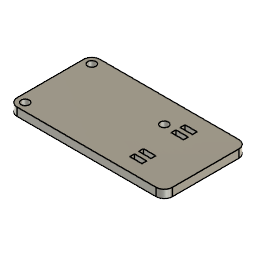
Arnes v1 (Autodesk Fusion 360 design; units mm, degrees)
Autodesk Fusion 360 part; units mm, degrees
(part 1 of 2)
sketch "Boceto1" plane through (0, 0, 0) normal (0, 0, 1) x (1, 0, 0)
  arc A0 (2, 20.32) -> (0, 18.32) centre (2, 18.32) ccw
  arc A1 (0, 2) -> (2, 0) centre (2, 2) ccw
  arc A2 (36.08, 0) -> (38.08, 2) centre (36.08, 2) ccw
  line L0 (38.08, 2) -> (38.08, 18.32)
  line L1 (36.08, 20.32) -> (2, 20.32)
  arc A3 (38.08, 18.32) -> (36.08, 20.32) centre (36.08, 18.32) ccw
  line L2 (2, 0) -> (36.08, 0)
  line L3 (0, 18.32) -> (0, 2)
  line L4 (25.2, 8.47, 1.57) -> (25.2, 7.99, 1.57)
  line L5 (25.2, 7.99, 1.57) -> (25.6, 7.99, 1.57)
  line L6 (25.6, 7.99, 1.57) -> (25.6, 8.47, 1.57)
  line L7 (25.6, 8.47, 1.57) -> (25.2, 8.47, 1.57)
  line L8 (25.2, 9.79, 1.57) -> (25.2, 9.31, 1.57)
  line L9 (25.6, 9.31, 1.57) -> (25.6, 9.79, 1.57)
  line L10 (25.6, 9.79, 1.57) -> (25.2, 9.79, 1.57)
  line L11 (25.2, 9.31, 1.57) -> (25.6, 9.31, 1.57)
  line L12 (24.511, 9.525, 1.57) -> (24.511, 7.9796, 1.57)
  line L13 (25.957, 8.1792, 1.57) -> (26.3634, 8.1792, 1.57)
  line L14 (25.957, 9.574, 1.57) -> (25.957, 8.1792, 1.57)
  line L15 (24.511, 7.9796, 1.57) -> (24.9174, 7.9796, 1.57)
  line L16 (26.3634, 9.574, 1.57) -> (25.957, 9.574, 1.57)
  line L17 (24.9174, 7.9796, 1.57) -> (24.9174, 9.525, 1.57)
  line L18 (26.3634, 8.1792, 1.57) -> (26.3634, 9.574, 1.57)
  line L19 (24.9174, 9.525, 1.57) -> (24.511, 9.525, 1.57)
  line L20 (25.85, 8.24, 1.571) -> (25.85, 9.54, 1.571)
  line L21 (24.95, 8.24, 1.571) -> (25.85, 8.24, 1.571)
  line L22 (24.95, 9.54, 1.571) -> (24.95, 8.24, 1.571)
  line L23 (25.85, 9.54, 1.571) -> (24.95, 8.24, 1.571)
  line L24 (25.85, 8.24, 1.571) -> (24.95, 9.54, 1.571)
  line L25 (25.85, 9.54, 1.571) -> (24.95, 9.54, 1.571)
  line L26 (25.4, 9.44, 1.72) -> (25.4, 9.44, 1.57)
  line L27 (25.4, 8.04, 1.57) -> (25.4, 8.04, 1.72)
  line L28 (25.4, 8.04, 1.72) -> (25.4, 8.34, 1.72)
  line L29 (25.4, 8.34, 1.72) -> (25.4, 8.34, 1.57)
  line L30 (25.4, 8.04, 1.72) -> (25.4, 8.34, 1.57)
  line L31 (25.4, 9.44, 1.57) -> (25.4, 9.74, 1.57)
  line L32 (25.4, 9.74, 1.57) -> (25.4, 9.74, 1.72)
  line L33 (25.4, 9.74, 1.72) -> (25.4, 9.44, 1.72)
  line L34 (25.4, 9.74, 1.72) -> (25.4, 9.44, 1.57)
  line L35 (25.4, 8.34, 1.57) -> (25.4, 8.04, 1.57)
  line L36 (25.4, 8.34, 1.72) -> (25.4, 8.04, 1.57)
  line L37 (25.4, 9.44, 1.72) -> (25.4, 9.74, 1.57)
  line L38 (25.02, 9.47, 2.27) -> (25.02, 9.21, 2.27)
  line L39 (25.4, 8.89, 2.27) -> (26.4, 8.89, 2.27)
  line L40 (25.78, 9.47, 2.27) -> (25.02, 9.47, 2.27)
  line L41 (25.02, 9.21, 2.27) -> (25.78, 9.21, 2.27)
  line L42 (25.78, 9.21, 2.27) -> (25.78, 9.47, 2.27)
  line L43 (25.4, 8.89, 2.27) -> (25.4, 7.89, 2.27)
  line L44 (22.21, 8.27, 1.57) -> (22.21, 7.43, 1.57)
  line L45 (22.21, 9.51, 1.57) -> (22.21, 10.35, 1.57)
  line L46 (23.51, 8.56, 1.57) -> (23.51, 9.22, 1.57)
  circle A4 through (25.56, 7.69, 1.57) (25.26, 7.8632, 1.57) (25.26, 7.5168, 1.57)
  line L47 (22.21, 10.35, 1.57) -> (22.985, 10.35, 1.57)
  line L48 (22.21, 7.43, 1.57) -> (22.985, 7.43, 1.57)
  arc A5 through (24.37, 8.24, 1.57) (24.3407, 8.3107, 1.57) (24.27, 8.34, 1.57)
  line L49 (24.37, 8.24, 1.57) -> (24.37, 7.64, 1.57)
  arc A6 through (24.37, 10.14, 1.57) (24.3407, 10.2107, 1.57) (24.27, 10.24, 1.57)
  arc A7 through (23.57, 10.24, 1.57) (23.4993, 10.2107, 1.57) (23.47, 10.14, 1.57)
  arc A8 through (23.47, 7.64, 1.57) (23.4993, 7.5693, 1.57) (23.57, 7.54, 1.57)
  arc A9 through (23.47, 9.54, 1.57) (23.4993, 9.4693, 1.57) (23.57, 9.44, 1.57)
  arc A10 through (24.27, 9.44, 1.57) (24.3407, 9.4693, 1.57) (24.37, 9.54, 1.57)
  line L50 (24.27, 10.24, 1.57) -> (23.57, 10.24, 1.57)
  line L51 (23.47, 8.24, 1.57) -> (23.47, 7.64, 1.57)
  line L52 (23.47, 10.14, 1.57) -> (23.47, 9.54, 1.57)
  line L53 (24.27, 9.44, 1.57) -> (23.57, 9.44, 1.57)
  line L54 (24.27, 7.54, 1.57) -> (23.57, 7.54, 1.57)
  arc A11 through (24.27, 7.54, 1.57) (24.3407, 7.5693, 1.57) (24.37, 7.64, 1.57)
  arc A12 through (23.57, 8.34, 1.57) (23.4993, 8.3107, 1.57) (23.47, 8.24, 1.57)
  line L55 (24.27, 8.34, 1.57) -> (23.57, 8.34, 1.57)
  line L56 (21.35, 9.19, 1.57) -> (21.35, 8.59, 1.57)
  arc A13 through (21.45, 9.29, 1.57) (21.3793, 9.2607, 1.57) (21.35, 9.19, 1.57)
  line L57 (22.15, 9.29, 1.57) -> (21.45, 9.29, 1.57)
  line L58 (22.15, 8.49, 1.57) -> (21.45, 8.49, 1.57)
  arc A14 through (22.15, 8.49, 1.57) (22.2207, 8.5193, 1.57) (22.25, 8.59, 1.57)
  arc A15 through (21.35, 8.59, 1.57) (21.3793, 8.5193, 1.57) (21.45, 8.49, 1.57)
  line L59 (22.25, 9.19, 1.57) -> (22.25, 8.59, 1.57)
  line L60 (24.37, 10.14, 1.57) -> (24.37, 9.54, 1.57)
  arc A16 through (22.25, 9.19, 1.57) (22.2207, 9.2607, 1.57) (22.15, 9.29, 1.57)
  line L61 (20.6856, 10.89, 1.57) -> (25.36, 10.89, 1.57)
  line L62 (21.0868, 5.62, 1.57) -> (25.36, 5.62, 1.57)
  line L63 (25.36, 12.16, 1.57) -> (20.6856, 12.16, 1.57)
  line L64 (25.36, 5.62, 1.57) -> (25.36, 6.89, 1.57)
  line L65 (20.6856, 12.16, 1.57) -> (20.6856, 10.89, 1.57)
  line L66 (25.36, 10.89, 1.57) -> (25.36, 12.16, 1.57)
  line L67 (25.36, 6.89, 1.57) -> (21.0868, 6.89, 1.57)
  line L68 (21.0868, 6.89, 1.57) -> (21.0868, 5.62, 1.57)
  circle A17 through (18.3, 11.415, 1.57) (18, 11.5882, 1.57) (18, 11.2418, 1.57)
  circle A18 through (18.3, 6.335, 1.57) (18, 6.5082, 1.57) (18, 6.1618, 1.57)
  line L69 (19.345, 9.54, 1.57) -> (19.345, 10.75, 1.57)
  line L70 (19.345, 14.62, 1.57) -> (19.345, 15.83, 1.57)
  line L71 (18.395, 9.54, 1.57) -> (18.395, 10.75, 1.57)
  line L72 (18.395, 14.62, 1.57) -> (18.395, 15.83, 1.57)
  line L73 (18.755, 15.83, 1.57) -> (18.755, 14.62, 1.57)
  line L74 (18.755, 10.75, 1.57) -> (18.755, 9.54, 1.57)
  line L75 (19.345, 7.03, 1.57) -> (19.345, 8.24, 1.57)
  line L76 (19.345, 12.11, 1.57) -> (19.345, 13.32, 1.57)
  line L77 (18.395, 7.03, 1.57) -> (18.395, 8.24, 1.57)
  line L78 (18.395, 12.11, 1.57) -> (18.395, 13.32, 1.57)
  line L79 (18.755, 13.32, 1.57) -> (18.755, 12.11, 1.57)
  line L80 (18.755, 8.24, 1.57) -> (18.755, 7.03, 1.57)
  line L81 (17.805, 9.54, 1.57) -> (18.395, 9.54, 1.57)
  line L82 (17.805, 14.62, 1.57) -> (18.395, 14.62, 1.57)
  line L83 (20.295, 10.75, 1.57) -> (19.705, 10.75, 1.57)
  line L84 (20.295, 15.83, 1.57) -> (19.705, 15.83, 1.57)
  line L85 (17.805, 13.32, 1.57) -> (17.805, 12.11, 1.57)
  line L86 (17.805, 8.24, 1.57) -> (17.805, 7.03, 1.57)
  line L87 (18.755, 12.11, 1.57) -> (19.345, 12.11, 1.57)
  line L88 (18.755, 7.03, 1.57) -> (19.345, 7.03, 1.57)
  line L89 (19.705, 7.03, 1.57) -> (20.295, 7.03, 1.57)
  line L90 (19.705, 12.11, 1.57) -> (20.295, 12.11, 1.57)
  line L91 (19.705, 14.62, 1.57) -> (20.295, 14.62, 1.57)
  line L92 (19.705, 9.54, 1.57) -> (20.295, 9.54, 1.57)
  line L93 (17.805, 7.03, 1.57) -> (18.395, 7.03, 1.57)
  line L94 (17.805, 12.11, 1.57) -> (18.395, 12.11, 1.57)
  line L95 (18.755, 9.54, 1.57) -> (19.345, 9.54, 1.57)
  line L96 (18.755, 14.62, 1.57) -> (19.345, 14.62, 1.57)
  line L97 (18.395, 13.32, 1.57) -> (17.805, 13.32, 1.57)
  line L98 (18.395, 8.24, 1.57) -> (17.805, 8.24, 1.57)
  line L99 (19.345, 13.32, 1.57) -> (18.755, 13.32, 1.57)
  line L100 (19.345, 8.24, 1.57) -> (18.755, 8.24, 1.57)
  line L101 (19.705, 8.24, 1.57) -> (19.705, 7.03, 1.57)
  line L102 (19.705, 13.32, 1.57) -> (19.705, 12.11, 1.57)
  line L103 (19.705, 15.83, 1.57) -> (19.705, 14.62, 1.57)
  line L104 (19.705, 10.75, 1.57) -> (19.705, 9.54, 1.57)
  line L105 (18.395, 15.83, 1.57) -> (17.805, 15.83, 1.57)
  line L106 (18.395, 10.75, 1.57) -> (17.805, 10.75, 1.57)
  line L107 (20.295, 12.11, 1.57) -> (20.295, 13.32, 1.57)
  line L108 (20.295, 7.03, 1.57) -> (20.295, 8.24, 1.57)
  line L109 (19.345, 10.75, 1.57) -> (18.755, 10.75, 1.57)
  line L110 (19.345, 15.83, 1.57) -> (18.755, 15.83, 1.57)
  line L111 (20.295, 8.24, 1.57) -> (19.705, 8.24, 1.57)
  line L112 (20.295, 13.32, 1.57) -> (19.705, 13.32, 1.57)
  line L113 (17.805, 15.83, 1.57) -> (17.805, 14.62, 1.57)
  line L114 (17.805, 10.75, 1.57) -> (17.805, 9.54, 1.57)
  line L115 (20.295, 9.54, 1.57) -> (20.295, 10.75, 1.57)
  line L116 (20.295, 14.62, 1.57) -> (20.295, 15.83, 1.57)
  line L117 (16.95, 11.1388, 1.57) -> (15.68, 11.1388, 1.57)
  line L118 (16.95, 16.2188, 1.57) -> (15.68, 16.2188, 1.57)
  line L119 (16.95, 6.78, 1.57) -> (16.95, 11.1388, 1.57)
  line L120 (16.95, 11.86, 1.57) -> (16.95, 16.2188, 1.57)
  line L121 (21.05, 6.78, 1.57) -> (22.32, 6.78, 1.57)
  line L122 (21.05, 11.86, 1.57) -> (22.32, 11.86, 1.57)
  line L123 (21.05, 16.6895, 1.57) -> (21.05, 11.86, 1.57)
  line L124 (21.05, 11.6095, 1.57) -> (21.05, 6.78, 1.57)
  line L125 (22.32, 11.86, 1.57) -> (22.32, 16.6895, 1.57)
  line L126 (22.32, 6.78, 1.57) -> (22.32, 11.6095, 1.57)
  line L127 (22.32, 16.6895, 1.57) -> (21.05, 16.6895, 1.57)
  line L128 (22.32, 11.6095, 1.57) -> (21.05, 11.6095, 1.57)
  line L129 (15.68, 16.2188, 1.57) -> (15.68, 11.86, 1.57)
  line L130 (15.68, 11.1388, 1.57) -> (15.68, 6.78, 1.57)
  line L131 (15.68, 6.78, 1.57) -> (16.95, 6.78, 1.57)
  line L132 (15.68, 11.86, 1.57) -> (16.95, 11.86, 1.57)
  line L133 (17.54, 14.82, 1.58) -> (17.54, 13.12, 1.58)
  line L134 (17.54, 9.74, 1.58) -> (17.54, 8.04, 1.58)
  line L135 (20.56, 8.04, 1.58) -> (20.56, 9.74, 1.58)
  line L136 (20.56, 13.12, 1.58) -> (20.56, 14.82, 1.58)
  line L137 (20.56, 9.74, 1.58) -> (17.54, 9.74, 1.58)
  line L138 (20.56, 14.82, 1.58) -> (17.54, 14.82, 1.58)
  line L139 (17.54, 14.82, 1.58) -> (20.56, 13.12, 1.58)
  line L140 (17.54, 9.74, 1.58) -> (20.56, 8.04, 1.58)
  line L141 (17.54, 8.04, 1.58) -> (20.56, 8.04, 1.58)
  line L142 (17.54, 13.12, 1.58) -> (20.56, 13.12, 1.58)
  line L143 (17.54, 13.12, 1.58) -> (20.56, 14.82, 1.58)
  line L144 (17.54, 8.04, 1.58) -> (20.56, 9.74, 1.58)
  line L145 (20, 13.05, 1.7) -> (20, 13.05, 2.0775)
  line L146 (20, 7.97, 1.7) -> (20, 7.97, 2.0775)
  line L147 (20, 7.44, 1.57) -> (20, 7.84, 1.57)
  line L148 (20, 12.52, 1.57) -> (20, 12.92, 1.57)
  line L149 (20, 13.0825, 2.11) -> (20, 13.12, 2.11)
  line L150 (20, 8.0025, 2.11) -> (20, 8.04, 2.11)
  arc A19 through (20, 12.92, 1.7325) (20, 12.9105, 1.7095) (20, 12.8875, 1.7)
  arc A20 through (20, 7.84, 1.7325) (20, 7.8305, 1.7095) (20, 7.8075, 1.7)
  line L151 (20, 8.04, 2.24) -> (20, 7.97, 2.24)
  line L152 (20, 13.12, 2.24) -> (20, 13.05, 2.24)
  arc A21 through (20, 7.84, 2.11) (20, 7.8781, 2.2019) (20, 7.97, 2.24)
  arc A22 through (20, 12.92, 2.11) (20, 12.9581, 2.2019) (20, 13.05, 2.24)
  arc A23 through (20, 7.97, 1.7) (20, 7.9319, 1.6081) (20, 7.84, 1.57)
  arc A24 through (20, 13.05, 1.7) (20, 13.0119, 1.6081) (20, 12.92, 1.57)
  arc A25 through (20, 13.05, 2.0775) (20, 13.0595, 2.1005) (20, 13.0825, 2.11)
  arc A26 through (20, 7.97, 2.0775) (20, 7.9795, 2.1005) (20, 8.0025, 2.11)
  line L153 (20, 7.8075, 1.7) -> (20, 7.44, 1.7)
  line L154 (20, 12.8875, 1.7) -> (20, 12.52, 1.7)
  line L155 (20, 13.12, 2.11) -> (20, 13.12, 2.24)
  line L156 (20, 8.04, 2.11) -> (20, 8.04, 2.24)
  line L157 (20, 12.92, 2.11) -> (20, 12.92, 1.7325)
  line L158 (20, 7.84, 2.11) -> (20, 7.84, 1.7325)
  line L159 (20, 7.44, 1.7) -> (20, 7.44, 1.57)
  line L160 (20, 12.52, 1.7) -> (20, 12.52, 1.57)
  line L161 (18.1, 7.44, 1.7) -> (18.1, 7.44, 1.57)
  line L162 (18.1, 12.52, 1.7) -> (18.1, 12.52, 1.57)
  arc A27 through (18.1, 7.84, 2.11) (18.1, 7.8781, 2.2019) (18.1, 7.97, 2.24)
  arc A28 through (18.1, 12.92, 2.11) (18.1, 12.9581, 2.2019) (18.1, 13.05, 2.24)
  arc A29 through (18.1, 7.97, 2.0775) (18.1, 7.9795, 2.1005) (18.1, 8.0025, 2.11)
  arc A30 through (18.1, 13.05, 2.0775) (18.1, 13.0595, 2.1005) (18.1, 13.0825, 2.11)
  arc A31 through (18.1, 13.05, 1.7) (18.1, 13.0119, 1.6081) (18.1, 12.92, 1.57)
  arc A32 through (18.1, 7.97, 1.7) (18.1, 7.9319, 1.6081) (18.1, 7.84, 1.57)
  line L163 (18.1, 13.12, 2.11) -> (18.1, 13.12, 2.24)
  line L164 (18.1, 8.04, 2.11) -> (18.1, 8.04, 2.24)
  line L165 (18.1, 7.44, 1.57) -> (18.1, 7.84, 1.57)
  line L166 (18.1, 12.52, 1.57) -> (18.1, 12.92, 1.57)
  line L167 (18.1, 12.8875, 1.7) -> (18.1, 12.52, 1.7)
  line L168 (18.1, 7.8075, 1.7) -> (18.1, 7.44, 1.7)
  line L169 (18.1, 7.97, 1.7) -> (18.1, 7.97, 2.0775)
  line L170 (18.1, 13.05, 1.7) -> (18.1, 13.05, 2.0775)
  line L171 (18.1, 12.92, 2.11) -> (18.1, 12.92, 1.7325)
  line L172 (18.1, 7.84, 2.11) -> (18.1, 7.84, 1.7325)
  arc A33 through (18.1, 7.84, 1.7325) (18.1, 7.8305, 1.7095) (18.1, 7.8075, 1.7)
  arc A34 through (18.1, 12.92, 1.7325) (18.1, 12.9105, 1.7095) (18.1, 12.8875, 1.7)
  line L173 (18.1, 8.04, 2.24) -> (18.1, 7.97, 2.24)
  line L174 (18.1, 13.12, 2.24) -> (18.1, 13.05, 2.24)
  line L175 (18.1, 8.0025, 2.11) -> (18.1, 8.04, 2.11)
  line L176 (18.1, 13.0825, 2.11) -> (18.1, 13.12, 2.11)
  circle A35 through (17.915, 13.41, 2.77) (17.7875, 13.4836, 2.77) (17.7875, 13.3364, 2.77)
  circle A36 through (17.915, 8.33, 2.77) (17.7875, 8.4036, 2.77) (17.7875, 8.2564, 2.77)
  circle A37 through (3.0505, 2, 1.57) (1.4748, 2.9098, 1.57) (1.4747, 1.0902, 1.57)
  circle A38 through (24.7675, 14.383, 1.57) (23.1918, 15.2928, 1.57) (23.1918, 13.4732, 1.57)
  circle A39 through (3.0505, 18.32, 1.57) (1.4748, 19.2298, 1.57) (1.4747, 17.4102, 1.57)
  circle A40 through (3, 18.32, 1.57) (1.5, 19.186, 1.57) (1.5, 17.454, 1.57)
  circle A41 through (24.717, 14.383, 1.57) (23.217, 15.249, 1.57) (23.217, 13.517, 1.57)
  circle A42 through (3, 2, 1.57) (1.5, 2.866, 1.57) (1.5, 1.134, 1.57)
  line L177 (20.32, 5.2437, 1.57) -> (20.32, 2.4975, 1.57)
  line L178 (13.97, 5.2437, 1.57) -> (13.97, 2.4975, 1.57)
  arc A43 through (14.643, 3.124, 1.57) (14.71, 3.0681, 1.57) (14.795, 3.048, 1.57)
  arc A44 through (20.993, 3.124, 1.57) (21.06, 3.0681, 1.57) (21.145, 3.048, 1.57)
  line L179 (14.795, 4.572, 1.57) -> (15.177, 4.572, 1.57)
  line L180 (21.145, 4.572, 1.57) -> (21.527, 4.572, 1.57)
  arc A45 through (14.795, 4.572, 1.57) (14.71, 4.5519, 1.57) (14.643, 4.496, 1.57)
  arc A46 through (21.145, 4.572, 1.57) (21.06, 4.5519, 1.57) (20.993, 4.496, 1.57)
  arc A47 through (19.113, 4.572, 1.57) (18.9786, 4.5164, 1.57) (18.923, 4.382, 1.57)
  arc A48 through (12.763, 4.572, 1.57) (12.6286, 4.5164, 1.57) (12.573, 4.382, 1.57)
  line L181 (15.367, 4.382, 1.57) -> (15.367, 3.238, 1.57)
  line L182 (21.717, 4.382, 1.57) -> (21.717, 3.238, 1.57)
  arc A49 through (12.573, 3.238, 1.57) (12.6286, 3.1036, 1.57) (12.763, 3.048, 1.57)
  arc A50 through (18.923, 3.238, 1.57) (18.9786, 3.1036, 1.57) (19.113, 3.048, 1.57)
  line L183 (20.355, 2.4975, 1.57) -> (20.355, 5.3201, 1.57)
  line L184 (14.005, 2.4975, 1.57) -> (14.005, 5.3201, 1.57)
  line L185 (13.386, 2.5285, 1.57) -> (13.386, 5.1174, 1.57)
  line L186 (19.736, 2.5285, 1.57) -> (19.736, 5.1174, 1.57)
  line L187 (14.047, 2.4347, 1.57) -> (14.047, 5.3687, 1.57)
  line L188 (20.397, 2.4347, 1.57) -> (20.397, 5.3687, 1.57)
  line L189 (15.177, 3.048, 1.57) -> (14.795, 3.048, 1.57)
  line L190 (21.527, 3.048, 1.57) -> (21.145, 3.048, 1.57)
  line L191 (14.047, 3.048, 1.57) -> (13.145, 3.048, 1.57)
  line L192 (20.397, 3.048, 1.57) -> (19.495, 3.048, 1.57)
  line L193 (19.736, 3.81, 1.57) -> (20.397, 4.572, 1.57)
  line L194 (13.386, 3.81, 1.57) -> (14.047, 4.572, 1.57)
  line L195 (20.397, 4.572, 1.57) -> (19.495, 4.572, 1.57)
  line L196 (14.047, 4.572, 1.57) -> (13.145, 4.572, 1.57)
  line L197 (22.2051, 3.81, 1.57) -> (18.3388, 3.81, 1.57)
  line L198 (15.8551, 3.81, 1.57) -> (11.9888, 3.81, 1.57)
  line L199 (19.113, 4.572, 1.57) -> (19.495, 4.572, 1.57)
  line L200 (12.763, 4.572, 1.57) -> (13.145, 4.572, 1.57)
  line L201 (14.005, 3.81, 1.57) -> (13.0185, 3.81, 1.57)
  line L202 (20.355, 3.81, 1.57) -> (19.3685, 3.81, 1.57)
  line L203 (14.986, 2.5853, 1.57) -> (14.986, 5.1016, 1.57)
  line L204 (21.336, 2.5853, 1.57) -> (21.336, 5.1016, 1.57)
  line L205 (15.367, 4.572, 1.57) -> (14.605, 3.048, 1.57)
  line L206 (21.717, 4.572, 1.57) -> (20.955, 3.048, 1.57)
  arc A51 through (21.527, 3.048, 1.57) (21.6614, 3.1036, 1.57) (21.717, 3.238, 1.57)
  arc A52 through (15.177, 3.048, 1.57) (15.3114, 3.1036, 1.57) (15.367, 3.238, 1.57)
  line L207 (14.005, 3.81, 1.57) -> (14.6606, 4.5164, 1.57)
  line L208 (20.355, 3.81, 1.57) -> (21.0106, 4.5164, 1.57)
  line L209 (12.573, 3.238, 1.57) -> (12.573, 4.382, 1.57)
  line L210 (18.923, 3.238, 1.57) -> (18.923, 4.382, 1.57)
  line L211 (20.355, 3.81, 1.57) -> (21.0106, 3.1036, 1.57)
  line L212 (14.005, 3.81, 1.57) -> (14.6606, 3.1036, 1.57)
  line L213 (13.386, 3.81, 1.57) -> (14.047, 3.048, 1.57)
  line L214 (19.736, 3.81, 1.57) -> (20.397, 3.048, 1.57)
  line L215 (20.955, 4.572, 1.57) -> (21.717, 3.048, 1.57)
  line L216 (14.605, 4.572, 1.57) -> (15.367, 3.048, 1.57)
  arc A53 through (21.717, 4.382, 1.57) (21.6614, 4.5164, 1.57) (21.527, 4.572, 1.57)
  arc A54 through (15.367, 4.382, 1.57) (15.3114, 4.5164, 1.57) (15.177, 4.572, 1.57)
  line L217 (19.495, 3.048, 1.57) -> (19.113, 3.048, 1.57)
  line L218 (13.145, 3.048, 1.57) -> (12.763, 3.048, 1.57)
  arc A55 through (21.717, 2.794, 1.57) (21.8966, 2.8684, 1.57) (21.971, 3.048, 1.57)
  arc A56 through (15.367, 2.794, 1.57) (15.5466, 2.8684, 1.57) (15.621, 3.048, 1.57)
  arc A57 through (21.971, 4.572, 1.57) (21.8966, 4.7516, 1.57) (21.717, 4.826, 1.57)
  arc A58 through (15.621, 4.572, 1.57) (15.5466, 4.7516, 1.57) (15.367, 4.826, 1.57)
  arc A59 through (18.923, 4.826, 1.57) (18.7434, 4.7516, 1.57) (18.669, 4.572, 1.57)
  arc A60 through (12.573, 4.826, 1.57) (12.3934, 4.7516, 1.57) (12.319, 4.572, 1.57)
  line L219 (18.669, 4.572, 1.57) -> (18.669, 3.048, 1.57)
  line L220 (12.319, 4.572, 1.57) -> (12.319, 3.048, 1.57)
  line L221 (15.367, 4.826, 1.57) -> (12.573, 4.826, 1.57)
  line L222 (21.717, 4.826, 1.57) -> (18.923, 4.826, 1.57)
  arc A61 through (18.669, 3.048, 1.57) (18.7434, 2.8684, 1.57) (18.923, 2.794, 1.57)
  arc A62 through (12.319, 3.048, 1.57) (12.3934, 2.8684, 1.57) (12.573, 2.794, 1.57)
  line L223 (18.923, 2.794, 1.57) -> (21.717, 2.794, 1.57)
  line L224 (12.573, 2.794, 1.57) -> (15.367, 2.794, 1.57)
  line L225 (21.971, 3.048, 1.57) -> (21.971, 4.572, 1.57)
  line L226 (15.621, 3.048, 1.57) -> (15.621, 4.572, 1.57)
  arc A63 through (20.955, 3.2385, 1.57) (21.0108, 3.1038, 1.57) (21.1455, 3.048, 1.57)
  arc A64 through (14.605, 3.2385, 1.57) (14.6608, 3.1038, 1.57) (14.7955, 3.048, 1.57)
  arc A65 through (21.717, 4.3815, 1.57) (21.6612, 4.5162, 1.57) (21.5265, 4.572, 1.57)
  arc A66 through (15.367, 4.3815, 1.57) (15.3112, 4.5162, 1.57) (15.1765, 4.572, 1.57)
  line L227 (19.685, 3.2385, 1.57) -> (19.685, 4.3815, 1.57)
  line L228 (13.335, 3.2385, 1.57) -> (13.335, 4.3815, 1.57)
  line L229 (15.367, 3.2385, 1.57) -> (15.367, 4.3815, 1.57)
  line L230 (21.717, 3.2385, 1.57) -> (21.717, 4.3815, 1.57)
  arc A67 through (19.4945, 3.048, 1.57) (19.6292, 3.1038, 1.57) (19.685, 3.2385, 1.57)
  arc A68 through (13.1445, 3.048, 1.57) (13.2792, 3.1038, 1.57) (13.335, 3.2385, 1.57)
  line L231 (19.1135, 3.048, 1.57) -> (19.4945, 3.048, 1.57)
  line L232 (12.7635, 3.048, 1.57) -> (13.1445, 3.048, 1.57)
  arc A69 through (21.5265, 3.048, 1.57) (21.6612, 3.1038, 1.57) (21.717, 3.2385, 1.57)
  arc A70 through (15.1765, 3.048, 1.57) (15.3112, 3.1038, 1.57) (15.367, 3.2385, 1.57)
  arc A71 through (21.1455, 4.572, 1.57) (21.0108, 4.5162, 1.57) (20.955, 4.3815, 1.57)
  arc A72 through (14.7955, 4.572, 1.57) (14.6608, 4.5162, 1.57) (14.605, 4.3815, 1.57)
  line L233 (19.1135, 4.572, 1.57) -> (19.4945, 4.572, 1.57)
  line L234 (12.7635, 4.572, 1.57) -> (13.1445, 4.572, 1.57)
  arc A73 through (12.7635, 4.572, 1.57) (12.6288, 4.5162, 1.57) (12.573, 4.3815, 1.57)
  arc A74 through (19.1135, 4.572, 1.57) (18.9788, 4.5162, 1.57) (18.923, 4.3815, 1.57)
  arc A75 through (13.335, 4.3815, 1.57) (13.2792, 4.5162, 1.57) (13.1445, 4.572, 1.57)
  arc A76 through (19.685, 4.3815, 1.57) (19.6292, 4.5162, 1.57) (19.4945, 4.572, 1.57)
  line L235 (18.923, 3.2385, 1.57) -> (18.923, 4.3815, 1.57)
  line L236 (12.573, 3.2385, 1.57) -> (12.573, 4.3815, 1.57)
  line L237 (14.7955, 4.572, 1.57) -> (15.1765, 4.572, 1.57)
  line L238 (21.1455, 4.572, 1.57) -> (21.5265, 4.572, 1.57)
  line L239 (14.7955, 3.048, 1.57) -> (15.1765, 3.048, 1.57)
  line L240 (21.1455, 3.048, 1.57) -> (21.5265, 3.048, 1.57)
  line L241 (14.605, 3.2385, 1.57) -> (14.605, 4.3815, 1.57)
  line L242 (20.955, 3.2385, 1.57) -> (20.955, 4.3815, 1.57)
  arc A77 through (12.573, 3.2385, 1.57) (12.6288, 3.1038, 1.57) (12.7635, 3.048, 1.57)
  arc A78 through (18.923, 3.2385, 1.57) (18.9788, 3.1038, 1.57) (19.1135, 3.048, 1.57)
  line L243 (18.8196, 5.0546, 1.57) -> (21.8204, 5.0546, 1.57)
  line L244 (12.4696, 5.0546, 1.57) -> (15.4704, 5.0546, 1.57)
  line L245 (12.5982, 1.7526, 1.57) -> (15.3418, 1.7526, 1.57)
  line L246 (18.9482, 1.7526, 1.57) -> (21.6918, 1.7526, 1.57)
  line L247 (21.8204, 5.8674, 1.57) -> (18.8196, 5.8674, 1.57)
  line L248 (15.4704, 5.8674, 1.57) -> (12.4696, 5.8674, 1.57)
  line L249 (21.6918, 1.7526, 1.57) -> (21.6918, 2.5654, 1.57)
  line L250 (15.3418, 1.7526, 1.57) -> (15.3418, 2.5654, 1.57)
  line L251 (18.8196, 5.8674, 1.57) -> (18.8196, 5.0546, 1.57)
  line L252 (12.4696, 5.8674, 1.57) -> (12.4696, 5.0546, 1.57)
  line L253 (15.4704, 5.0546, 1.57) -> (15.4704, 5.8674, 1.57)
  line L254 (21.8204, 5.0546, 1.57) -> (21.8204, 5.8674, 1.57)
  line L255 (15.3418, 2.5654, 1.57) -> (12.5982, 2.5654, 1.57)
  line L256 (21.6918, 2.5654, 1.57) -> (18.9482, 2.5654, 1.57)
  line L257 (12.5982, 2.5654, 1.57) -> (12.5982, 1.7526, 1.57)
  line L258 (18.9482, 2.5654, 1.57) -> (18.9482, 1.7526, 1.57)
  line L259 (27.94, 19.2664, 1.57) -> (33.0454, 19.2664, 1.57)
  line L260 (27.94, 9.1064, 1.57) -> (33.0454, 9.1064, 1.57)
  line L261 (29.21, 6.9764, 1.57) -> (29.21, 7.684, 1.57)
  line L262 (29.21, 17.1364, 1.57) -> (29.21, 17.844, 1.57)
  line L263 (36.83, 13.3147, 1.57) -> (36.83, 17.2183, 1.57)
  line L264 (36.83, 3.1547, 1.57) -> (36.83, 7.0583, 1.57)
  line L265 (33.02, 11.24, 1.57) -> (27.94, 11.24, 1.57)
  line L266 (33.02, 1.08, 1.57) -> (27.94, 1.08, 1.57)
  line L267 (27.94, 12.51, 1.57) -> (29.21, 12.51, 1.57)
  line L268 (27.94, 2.35, 1.57) -> (29.21, 2.35, 1.57)
  line L269 (29.21, 2.35, 1.57) -> (29.21, 2.9909, 1.57)
  line L270 (29.21, 12.51, 1.57) -> (29.21, 13.1509, 1.57)
  line L271 (27.94, 11.24, 1.57) -> (27.94, 12.51, 1.57)
  line L272 (27.94, 1.08, 1.57) -> (27.94, 2.35, 1.57)
  line L273 (27.94, 17.844, 1.57) -> (27.94, 19.2664, 1.57)
  line L274 (27.94, 7.684, 1.57) -> (27.94, 9.1064, 1.57)
  line L275 (29.21, 7.684, 1.57) -> (27.94, 7.684, 1.57)
  line L276 (29.21, 17.844, 1.57) -> (27.94, 17.844, 1.57)
  line L277 (36.87, 2.705, 1.57) -> (33.19, 2.705, 1.57)
  line L278 (36.87, 12.865, 1.57) -> (33.19, 12.865, 1.57)
  line L279 (29.33, 4.455, 1.57) -> (26.33, 4.455, 1.57)
  line L280 (29.33, 14.615, 1.57) -> (26.33, 14.615, 1.57)
  line L281 (29.33, 6.655, 1.57) -> (26.33, 6.655, 1.57)
  line L282 (29.33, 16.815, 1.57) -> (26.33, 16.815, 1.57)
  line L283 (33.19, 1.055, 1.57) -> (36.87, 1.055, 1.57)
  line L284 (33.19, 11.215, 1.57) -> (36.87, 11.215, 1.57)
  line L285 (26.33, 14.615, 1.57) -> (26.33, 13.465, 1.57)
  line L286 (26.33, 4.455, 1.57) -> (26.33, 3.305, 1.57)
  line L287 (26.33, 5.505, 1.57) -> (29.33, 5.505, 1.57)
  line L288 (26.33, 15.665, 1.57) -> (29.33, 15.665, 1.57)
  line L289 (36.87, 7.455, 1.57) -> (36.87, 9.105, 1.57)
  line L290 (36.87, 17.615, 1.57) -> (36.87, 19.265, 1.57)
  line L291 (26.33, 3.305, 1.57) -> (29.33, 3.305, 1.57)
  line L292 (26.33, 13.465, 1.57) -> (29.33, 13.465, 1.57)
  line L293 (36.87, 11.215, 1.57) -> (36.87, 12.865, 1.57)
  line L294 (36.87, 1.055, 1.57) -> (36.87, 2.705, 1.57)
  line L295 (29.33, 15.665, 1.57) -> (29.33, 16.815, 1.57)
  line L296 (29.33, 5.505, 1.57) -> (29.33, 6.655, 1.57)
  line L297 (26.33, 16.815, 1.57) -> (26.33, 15.665, 1.57)
  line L298 (26.33, 6.655, 1.57) -> (26.33, 5.505, 1.57)
  line L299 (33.19, 12.865, 1.57) -> (33.19, 11.215, 1.57)
  line L300 (33.19, 2.705, 1.57) -> (33.19, 1.055, 1.57)
  line L301 (33.19, 7.455, 1.57) -> (36.87, 7.455, 1.57)
  line L302 (33.19, 17.615, 1.57) -> (36.87, 17.615, 1.57)
  line L303 (29.33, 13.465, 1.57) -> (29.33, 14.615, 1.57)
  line L304 (29.33, 3.305, 1.57) -> (29.33, 4.455, 1.57)
  line L305 (36.87, 9.105, 1.57) -> (33.19, 9.105, 1.57)
  line L306 (36.87, 19.265, 1.57) -> (33.19, 19.265, 1.57)
  line L307 (33.19, 19.265, 1.57) -> (33.19, 17.615, 1.57)
  line L308 (33.19, 9.105, 1.57) -> (33.19, 7.455, 1.57)
  line L309 (39.37, 5.08, 1.57) -> (40.64, 5.08, 1.57)
  line L310 (39.37, 15.24, 1.57) -> (40.64, 15.24, 1.57)
  line L311 (38.1, 9.3532, 1.57) -> (38.1, 5.08, 1.57)
  line L312 (38.1, 19.5132, 1.57) -> (38.1, 15.24, 1.57)
  line L313 (39.37, 9.3532, 1.57) -> (38.1, 9.3532, 1.57)
  line L314 (39.37, 19.5132, 1.57) -> (38.1, 19.5132, 1.57)
  line L315 (40.64, 5.08, 1.57) -> (40.64, 9.7544, 1.57)
  line L316 (40.64, 15.24, 1.57) -> (40.64, 19.9144, 1.57)
  line L317 (40.64, 9.7544, 1.57) -> (39.37, 9.7544, 1.57)
  line L318 (40.64, 19.9144, 1.57) -> (39.37, 19.9144, 1.57)
  line L319 (39.37, 19.9144, 1.57) -> (39.37, 15.24, 1.57)
  line L320 (39.37, 9.7544, 1.57) -> (39.37, 5.08, 1.57)
  line L321 (39.37, 5.08, 1.57) -> (39.37, 9.3532, 1.57)
  line L322 (39.37, 15.24, 1.57) -> (39.37, 19.5132, 1.57)
  line L323 (38.1, 5.08, 1.57) -> (39.37, 5.08, 1.57)
  line L324 (38.1, 15.24, 1.57) -> (39.37, 15.24, 1.57)
  line L325 (5.42, 5.84, 1.57) -> (3.62, 5.84, 1.57)
  line L326 (5.42, 14.48, 1.57) -> (3.62, 14.48, 1.57)
  line L327 (6.78, 11.06, 1.57) -> (6.78, 10.76, 1.57)
  line L328 (6.78, 8.01, 1.57) -> (6.78, 7.41, 1.57)
  line L329 (7.78, 10.76, 1.57) -> (7.78, 11.06, 1.57)
  line L330 (7.78, 12.91, 1.57) -> (6.78, 12.91, 1.57)
  line L331 (6.78, 12.91, 1.57) -> (6.78, 12.31, 1.57)
  line L332 (6.78, 9.26, 1.57) -> (7.78, 9.26, 1.57)
  line L333 (7.78, 13.085, 1.57) -> (7.78, 13.685, 1.57)
  line L334 (6.78, 12.31, 1.57) -> (7.78, 12.31, 1.57)
  line L335 (6.78, 6.635, 1.57) -> (7.78, 6.635, 1.57)
  line L336 (7.78, 9.06, 1.57) -> (6.78, 9.06, 1.57)
  line L337 (7.78, 11.76, 1.57) -> (7.78, 12.06, 1.57)
  line L338 (6.78, 10.06, 1.57) -> (6.78, 9.76, 1.57)
  line L339 (7.78, 12.31, 1.57) -> (7.78, 12.91, 1.57)
  line L340 (6.78, 9.76, 1.57) -> (7.78, 9.76, 1.57)
  line L341 (7.78, 10.06, 1.57) -> (6.78, 10.06, 1.57)
  line L342 (6.78, 7.235, 1.57) -> (6.78, 6.635, 1.57)
  line L343 (6.78, 8.26, 1.57) -> (7.78, 8.26, 1.57)
  line L344 (7.78, 8.26, 1.57) -> (7.78, 8.56, 1.57)
  line L345 (6.78, 9.06, 1.57) -> (6.78, 8.76, 1.57)
  line L346 (6.78, 8.76, 1.57) -> (7.78, 8.76, 1.57)
  line L347 (7.78, 9.76, 1.57) -> (7.78, 10.06, 1.57)
  line L348 (6.78, 10.56, 1.57) -> (6.78, 10.26, 1.57)
  line L349 (6.78, 7.41, 1.57) -> (7.78, 7.41, 1.57)
  line L350 (7.78, 7.235, 1.57) -> (6.78, 7.235, 1.57)
  line L351 (7.78, 6.635, 1.57) -> (7.78, 7.235, 1.57)
  line L352 (7.78, 7.41, 1.57) -> (7.78, 8.01, 1.57)
  line L353 (7.78, 8.01, 1.57) -> (6.78, 8.01, 1.57)
  line L354 (7.78, 8.76, 1.57) -> (7.78, 9.06, 1.57)
  line L355 (6.78, 9.56, 1.57) -> (6.78, 9.26, 1.57)
  line L356 (7.78, 9.56, 1.57) -> (6.78, 9.56, 1.57)
  line L357 (7.78, 8.56, 1.57) -> (6.78, 8.56, 1.57)
  line L358 (7.78, 11.06, 1.57) -> (6.78, 11.06, 1.57)
  line L359 (6.78, 10.76, 1.57) -> (7.78, 10.76, 1.57)
  line L360 (7.78, 10.26, 1.57) -> (7.78, 10.56, 1.57)
  line L361 (7.78, 10.56, 1.57) -> (6.78, 10.56, 1.57)
  line L362 (7.78, 9.26, 1.57) -> (7.78, 9.56, 1.57)
  line L363 (6.78, 10.26, 1.57) -> (7.78, 10.26, 1.57)
  line L364 (7.78, 13.685, 1.57) -> (6.78, 13.685, 1.57)
  line L365 (6.78, 8.56, 1.57) -> (6.78, 8.26, 1.57)
  line L366 (6.78, 13.685, 1.57) -> (6.78, 13.085, 1.57)
  line L367 (6.78, 13.085, 1.57) -> (7.78, 13.085, 1.57)
  line L368 (6.78, 12.06, 1.57) -> (6.78, 11.76, 1.57)
  line L369 (6.78, 11.26, 1.57) -> (7.78, 11.26, 1.57)
  line L370 (6.78, 11.76, 1.57) -> (7.78, 11.76, 1.57)
  line L371 (6.78, 11.56, 1.57) -> (6.78, 11.26, 1.57)
  arc A79 through (7.005, 5.542, 1.57) (7.305, 5.842, 1.57) (7.005, 6.142, 1.57)
  circle A80 through (2.725, 5.842, 1.57) (2.425, 6.0152, 1.57) (2.425, 5.6688, 1.57)
  circle A81 through (6.905, 14.478, 1.57) (6.605, 14.6512, 1.57) (6.605, 14.3048, 1.57)
  circle A82 through (6.905, 5.842, 1.57) (6.605, 6.0152, 1.57) (6.605, 5.6688, 1.57)
  line L372 (7.005, 14.778, 1.57) -> (6.405, 14.778, 1.57)
  arc A83 through (2.825, 14.178, 1.57) (3.125, 14.478, 1.57) (2.825, 14.778, 1.57)
  line L373 (6.405, 14.178, 1.57) -> (7.005, 14.178, 1.57)
  line L374 (7.005, 6.142, 1.57) -> (6.405, 6.142, 1.57)
  arc A84 through (2.225, 14.778, 1.57) (1.925, 14.478, 1.57) (2.225, 14.178, 1.57)
  arc A85 through (2.825, 5.542, 1.57) (3.125, 5.842, 1.57) (2.825, 6.142, 1.57)
  line L375 (6.405, 5.542, 1.57) -> (7.005, 5.542, 1.57)
  line L376 (2.225, 14.178, 1.57) -> (2.825, 14.178, 1.57)
  line L377 (7.78, 11.56, 1.57) -> (6.78, 11.56, 1.57)
  line L378 (2.825, 14.778, 1.57) -> (2.225, 14.778, 1.57)
  line L379 (2.225, 5.542, 1.57) -> (2.825, 5.542, 1.57)
  line L380 (7.78, 11.26, 1.57) -> (7.78, 11.56, 1.57)
  circle A86 through (2.725, 14.478, 1.57) (2.425, 14.6512, 1.57) (2.425, 14.3048, 1.57)
  arc A87 through (7.005, 14.178, 1.57) (7.305, 14.478, 1.57) (7.005, 14.778, 1.57)
  line L381 (2.825, 6.142, 1.57) -> (2.225, 6.142, 1.57)
  arc A88 through (2.225, 6.142, 1.57) (1.925, 5.842, 1.57) (2.225, 5.542, 1.57)
  arc A89 through (6.405, 14.778, 1.57) (6.105, 14.478, 1.57) (6.405, 14.178, 1.57)
  line L382 (7.78, 12.06, 1.57) -> (6.78, 12.06, 1.57)
  arc A90 through (6.405, 6.142, 1.57) (6.105, 5.842, 1.57) (6.405, 5.542, 1.57)
  line L383 (4.699, 8.9578, 1.57) -> (5.461, 8.9578, 1.57)
  line L384 (5.461, 8.9578, 1.57) -> (5.461, 11.3622, 1.57)
  line L385 (4.699, 11.3622, 1.57) -> (4.699, 8.9578, 1.57)
  line L386 (3.429, 9.028, 1.57) -> (4.191, 9.028, 1.57)
  line L387 (4.191, 9.028, 1.57) -> (4.191, 11.292, 1.57)
  line L388 (4.191, 11.292, 1.57) -> (3.429, 11.292, 1.57)
  line L389 (5.461, 11.3622, 1.57) -> (4.699, 11.3622, 1.57)
  line L390 (3.429, 11.292, 1.57) -> (3.429, 9.028, 1.57)
  circle A91 through (6.5, 7.27, 1.57) (6.0125, 7.5515, 1.57) (6.0125, 6.9885, 1.57)
  circle A92 through (6.5, 13.05, 1.57) (6.0125, 13.3315, 1.57) (6.0125, 12.7685, 1.57)
  line L391 (2.84, 14.478, 1.57) -> (2.22, 14.478, 1.57)
  line L392 (7.255, 5.842, 1.57) -> (6.155, 5.842, 1.57)
  line L393 (7.255, 14.478, 1.57) -> (6.155, 14.478, 1.57)
  line L394 (2.84, 5.842, 1.57) -> (2.22, 5.842, 1.57)
  circle A93 through (15.62, 10.79, 1.57) (15.245, 11.0065, 1.57) (15.245, 10.5735, 1.57)
  line L395 (14.57, 10.79, 1.57) -> (14.57, 9.99, 1.57)
  line L396 (14.57, 9.99, 1.57) -> (14.87, 9.99, 1.57)
  line L397 (13.57, 9.99, 1.57) -> (13.87, 9.99, 1.57)
  line L398 (15.22, 9.79, 1.57) -> (12.72, 9.79, 1.57)
  line L399 (14.57, 7.79, 1.57) -> (14.57, 6.99, 1.57)
  line L400 (13.87, 6.99, 1.57) -> (13.87, 7.79, 1.57)
  line L401 (13.07, 10.79, 1.57) -> (13.07, 9.99, 1.57)
  line L402 (12.72, 7.99, 1.57) -> (15.22, 7.99, 1.57)
  line L403 (13.37, 7.79, 1.57) -> (13.07, 7.79, 1.57)
  line L404 (14.07, 9.99, 1.57) -> (14.37, 9.99, 1.57)
  line L405 (14.37, 7.79, 1.57) -> (14.07, 7.79, 1.57)
  line L406 (13.37, 6.99, 1.57) -> (13.37, 7.79, 1.57)
  line L407 (14.37, 10.79, 1.57) -> (14.07, 10.79, 1.57)
  line L408 (12.72, 9.79, 1.57) -> (12.72, 7.99, 1.57)
  line L409 (13.87, 7.79, 1.57) -> (13.57, 7.79, 1.57)
  line L410 (13.07, 7.79, 1.57) -> (13.07, 6.99, 1.57)
  line L411 (14.37, 6.99, 1.57) -> (14.37, 7.79, 1.57)
  line L412 (14.87, 7.79, 1.57) -> (14.57, 7.79, 1.57)
  line L413 (13.57, 6.99, 1.57) -> (13.87, 6.99, 1.57)
  line L414 (13.37, 10.79, 1.57) -> (13.07, 10.79, 1.57)
  line L415 (14.07, 10.79, 1.57) -> (14.07, 9.99, 1.57)
  line L416 (14.87, 9.99, 1.57) -> (14.87, 10.79, 1.57)
  line L417 (13.07, 9.99, 1.57) -> (13.37, 9.99, 1.57)
  line L418 (14.07, 7.79, 1.57) -> (14.07, 6.99, 1.57)
  line L419 (15.22, 7.99, 1.57) -> (15.22, 9.79, 1.57)
  line L420 (13.57, 7.79, 1.57) -> (13.57, 6.99, 1.57)
  line L421 (13.37, 9.99, 1.57) -> (13.37, 10.79, 1.57)
  line L422 (13.87, 10.79, 1.57) -> (13.57, 10.79, 1.57)
  line L423 (14.37, 9.99, 1.57) -> (14.37, 10.79, 1.57)
  line L424 (14.07, 6.99, 1.57) -> (14.37, 6.99, 1.57)
  line L425 (14.57, 6.99, 1.57) -> (14.87, 6.99, 1.57)
  line L426 (13.57, 10.79, 1.57) -> (13.57, 9.99, 1.57)
  line L427 (13.87, 9.99, 1.57) -> (13.87, 10.79, 1.57)
  line L428 (14.87, 6.99, 1.57) -> (14.87, 7.79, 1.57)
  line L429 (13.07, 6.99, 1.57) -> (13.37, 6.99, 1.57)
  line L430 (14.87, 10.79, 1.57) -> (14.57, 10.79, 1.57)
  line L431 (10.795, 11.3047, 1.57) -> (10.795, 6.4753, 1.57)
  line L432 (12.065, 11.3047, 1.57) -> (10.795, 11.3047, 1.57)
  line L433 (15.875, 11.0694, 1.57) -> (15.875, 6.7106, 1.57)
  line L434 (10.795, 6.4753, 1.57) -> (12.065, 6.4753, 1.57)
  line L435 (17.145, 11.0694, 1.57) -> (15.875, 11.0694, 1.57)
  line L436 (17.145, 6.7106, 1.57) -> (17.145, 11.0694, 1.57)
  line L437 (15.875, 6.7106, 1.57) -> (17.145, 6.7106, 1.57)
  line L438 (12.065, 6.4753, 1.57) -> (12.065, 11.3047, 1.57)
  circle A94 through (15.12, 16.525, 1.57) (14.82, 16.6982, 1.57) (14.82, 16.3518, 1.57)
  line L439 (13.675, 14.62, 1.57) -> (14.265, 14.62, 1.57)
  line L440 (14.265, 14.62, 1.57) -> (14.265, 15.83, 1.57)
  line L441 (14.265, 15.83, 1.57) -> (13.675, 15.83, 1.57)
  line L442 (14.625, 15.83, 1.57) -> (14.625, 14.62, 1.57)
  line L443 (15.215, 14.62, 1.57) -> (15.215, 15.83, 1.57)
  line L444 (12.725, 15.83, 1.57) -> (12.725, 14.62, 1.57)
  line L445 (12.725, 14.62, 1.57) -> (13.315, 14.62, 1.57)
  line L446 (13.315, 14.62, 1.57) -> (13.315, 15.83, 1.57)
  line L447 (13.315, 15.83, 1.57) -> (12.725, 15.83, 1.57)
  line L448 (12.725, 13.32, 1.57) -> (12.725, 12.11, 1.57)
  line L449 (12.725, 12.11, 1.57) -> (13.315, 12.11, 1.57)
  line L450 (13.315, 12.11, 1.57) -> (13.315, 13.32, 1.57)
  line L451 (13.315, 13.32, 1.57) -> (12.725, 13.32, 1.57)
  line L452 (14.625, 13.32, 1.57) -> (14.625, 12.11, 1.57)
  line L453 (14.625, 12.11, 1.57) -> (15.215, 12.11, 1.57)
  line L454 (14.625, 14.62, 1.57) -> (15.215, 14.62, 1.57)
  line L455 (15.215, 15.83, 1.57) -> (14.625, 15.83, 1.57)
  line L456 (13.675, 15.83, 1.57) -> (13.675, 14.62, 1.57)
  line L457 (14.265, 13.32, 1.57) -> (13.675, 13.32, 1.57)
  line L458 (15.215, 13.32, 1.57) -> (14.625, 13.32, 1.57)
  line L459 (14.265, 12.11, 1.57) -> (14.265, 13.32, 1.57)
  line L460 (15.215, 12.11, 1.57) -> (15.215, 13.32, 1.57)
  line L461 (13.675, 12.11, 1.57) -> (14.265, 12.11, 1.57)
  line L462 (13.675, 13.32, 1.57) -> (13.675, 12.11, 1.57)
  line L463 (16.07, 11.7212, 1.57) -> (17.34, 11.7212, 1.57)
  line L464 (10.7, 16.08, 1.57) -> (10.7, 11.2505, 1.57)
  line L465 (11.97, 11.2505, 1.57) -> (11.97, 16.08, 1.57)
  line L466 (10.7, 11.2505, 1.57) -> (11.97, 11.2505, 1.57)
  line L467 (11.97, 16.08, 1.57) -> (10.7, 16.08, 1.57)
  line L468 (17.34, 11.7212, 1.57) -> (17.34, 16.08, 1.57)
  line L469 (17.34, 16.08, 1.57) -> (16.07, 16.08, 1.57)
  line L470 (16.07, 16.08, 1.57) -> (16.07, 11.7212, 1.57)
  line L471 (12.46, 14.82, 1.58) -> (12.46, 13.12, 1.58)
  line L472 (15.48, 14.82, 1.58) -> (12.46, 13.12, 1.58)
  line L473 (15.48, 13.12, 1.58) -> (12.46, 14.82, 1.58)
  line L474 (15.48, 13.12, 1.58) -> (15.48, 14.82, 1.58)
  line L475 (15.48, 14.82, 1.58) -> (12.46, 14.82, 1.58)
  line L476 (12.46, 13.12, 1.58) -> (15.48, 13.12, 1.58)
  line L477 (13.02, 14.82, 2.24) -> (13.02, 14.89, 2.24)
  line L478 (13.02, 15.42, 1.57) -> (13.02, 15.02, 1.57)
  line L479 (13.02, 14.82, 2.11) -> (13.02, 14.82, 2.24)
  arc A95 through (13.02, 15.02, 2.11) (13.02, 14.9819, 2.2019) (13.02, 14.89, 2.24)
  arc A96 through (13.02, 15.02, 1.7325) (13.02, 15.0295, 1.7095) (13.02, 15.0525, 1.7)
  line L480 (13.02, 15.42, 1.7) -> (13.02, 15.42, 1.57)
  arc A97 through (13.02, 14.89, 1.7) (13.02, 14.9281, 1.6081) (13.02, 15.02, 1.57)
  line L481 (13.02, 14.8575, 2.11) -> (13.02, 14.82, 2.11)
  line L482 (13.02, 15.0525, 1.7) -> (13.02, 15.42, 1.7)
  line L483 (13.02, 14.89, 1.7) -> (13.02, 14.89, 2.0775)
  line L484 (13.02, 15.02, 2.11) -> (13.02, 15.02, 1.7325)
  arc A98 through (13.02, 14.89, 2.0775) (13.02, 14.8805, 2.1005) (13.02, 14.8575, 2.11)
  arc A99 through (14.92, 15.02, 1.7325) (14.92, 15.0295, 1.7095) (14.92, 15.0525, 1.7)
  line L485 (14.92, 15.42, 1.57) -> (14.92, 15.02, 1.57)
  arc A100 through (14.92, 14.89, 1.7) (14.92, 14.9281, 1.6081) (14.92, 15.02, 1.57)
  line L486 (14.92, 15.0525, 1.7) -> (14.92, 15.42, 1.7)
  line L487 (14.92, 14.89, 1.7) -> (14.92, 14.89, 2.0775)
  line L488 (14.92, 14.82, 2.24) -> (14.92, 14.89, 2.24)
  line L489 (14.92, 15.02, 2.11) -> (14.92, 15.02, 1.7325)
  line L490 (14.92, 14.82, 2.11) -> (14.92, 14.82, 2.24)
  arc A101 through (14.92, 14.89, 2.0775) (14.92, 14.8805, 2.1005) (14.92, 14.8575, 2.11)
  arc A102 through (14.92, 15.02, 2.11) (14.92, 14.9819, 2.2019) (14.92, 14.89, 2.24)
  line L491 (14.92, 15.42, 1.7) -> (14.92, 15.42, 1.57)
  line L492 (14.92, 14.8575, 2.11) -> (14.92, 14.82, 2.11)
  circle A103 through (15.275, 14.53, 2.77) (15.1475, 14.6036, 2.77) (15.1475, 14.4564, 2.77)
  line L493 (10.46, 5.53, 1.57) -> (10.46, 4.63, 1.57)
  line L494 (9.86, 3.36, 1.57) -> (9.86, 4.26, 1.57)
  line L495 (10.46, 10.61, 1.57) -> (10.46, 9.71, 1.57)
  line L496 (11.16, 9.71, 1.57) -> (11.16, 10.61, 1.57)
  line L497 (9.16, 4.26, 1.57) -> (9.16, 3.36, 1.57)
  line L498 (11.16, 4.63, 1.57) -> (11.16, 5.53, 1.57)
  line L499 (9.86, 5.53, 1.57) -> (9.16, 5.53, 1.57)
  line L500 (10.46, 3.36, 1.57) -> (11.16, 3.36, 1.57)
  line L501 (9.86, 10.61, 1.57) -> (9.16, 10.61, 1.57)
  line L502 (9.16, 9.71, 1.57) -> (9.86, 9.71, 1.57)
  line L503 (11.16, 4.26, 1.57) -> (10.46, 4.26, 1.57)
  line L504 (9.16, 4.63, 1.57) -> (9.86, 4.63, 1.57)
  line L505 (10.46, 4.26, 1.57) -> (10.46, 3.36, 1.57)
  line L506 (9.86, 4.63, 1.57) -> (9.86, 5.53, 1.57)
  line L507 (9.86, 9.71, 1.57) -> (9.86, 10.61, 1.57)
  line L508 (9.16, 10.61, 1.57) -> (9.16, 9.71, 1.57)
  line L509 (9.16, 5.53, 1.57) -> (9.16, 4.63, 1.57)
  line L510 (11.16, 3.36, 1.57) -> (11.16, 4.26, 1.57)
  line L511 (9.86, 4.26, 1.57) -> (9.16, 4.26, 1.57)
  line L512 (10.46, 4.63, 1.57) -> (11.16, 4.63, 1.57)
  line L513 (10.46, 9.71, 1.57) -> (11.16, 9.71, 1.57)
  line L514 (11.16, 10.61, 1.57) -> (10.46, 10.61, 1.57)
  line L515 (11.16, 5.53, 1.57) -> (10.46, 5.53, 1.57)
  line L516 (9.16, 3.36, 1.57) -> (9.86, 3.36, 1.57)
  line L517 (9.525, 5.842, 1.57) -> (13.8838, 5.842, 1.57)
  line L518 (9.525, 10.922, 1.57) -> (13.8838, 10.922, 1.57)
  line L519 (10.795, 3.048, 1.57) -> (6.4362, 3.048, 1.57)
  line L520 (13.8838, 5.842, 1.57) -> (13.8838, 7.112, 1.57)
  line L521 (6.4362, 3.048, 1.57) -> (6.4362, 1.778, 1.57)
  line L522 (13.8838, 10.922, 1.57) -> (13.8838, 12.192, 1.57)
  line L523 (13.8838, 12.192, 1.57) -> (9.525, 12.192, 1.57)
  line L524 (6.4362, 1.778, 1.57) -> (10.795, 1.778, 1.57)
  line L525 (13.8838, 7.112, 1.57) -> (9.525, 7.112, 1.57)
  line L526 (9.525, 12.192, 1.57) -> (9.525, 10.922, 1.57)
  line L527 (9.525, 7.112, 1.57) -> (9.525, 5.842, 1.57)
  line L528 (10.795, 1.778, 1.57) -> (10.795, 3.048, 1.57)
  line L529 (9.525, 3.175, 1.57) -> (14.3545, 3.175, 1.57)
  line L530 (10.795, 5.715, 1.57) -> (5.9655, 5.715, 1.57)
  line L531 (9.525, 8.255, 1.57) -> (14.3545, 8.255, 1.57)
  line L532 (5.9655, 5.715, 1.57) -> (5.9655, 4.445, 1.57)
  line L533 (14.3545, 8.255, 1.57) -> (14.3545, 9.525, 1.57)
  line L534 (14.3545, 3.175, 1.57) -> (14.3545, 4.445, 1.57)
  line L535 (14.3545, 9.525, 1.57) -> (9.525, 9.525, 1.57)
  line L536 (14.3545, 4.445, 1.57) -> (9.525, 4.445, 1.57)
  line L537 (5.9655, 4.445, 1.57) -> (10.795, 4.445, 1.57)
  line L538 (10.795, 4.445, 1.57) -> (10.795, 5.715, 1.57)
  line L539 (9.525, 9.525, 1.57) -> (9.525, 8.255, 1.57)
  line L540 (9.525, 4.445, 1.57) -> (9.525, 3.175, 1.57)
  line L541 (10.685, 5.355, 1.57) -> (9.635, 4.805, 1.57)
  line L542 (10.685, 10.435, 1.57) -> (9.635, 9.885, 1.57)
  line L543 (9.635, 3.535, 1.57) -> (10.685, 4.085, 1.57)
  line L544 (9.635, 3.535, 1.57) -> (10.685, 3.535, 1.57)
  line L545 (10.685, 10.435, 1.57) -> (9.635, 10.435, 1.57)
  line L546 (10.685, 5.355, 1.57) -> (9.635, 5.355, 1.57)
  line L547 (9.885, 3.535, 1.57) -> (9.885, 4.085, 1.57)
  line L548 (10.435, 5.355, 1.57) -> (10.435, 4.805, 1.57)
  line L549 (10.435, 10.435, 1.57) -> (10.435, 9.885, 1.57)
  line L550 (9.635, 4.085, 1.57) -> (9.635, 3.535, 1.57)
  line L551 (10.685, 4.805, 1.57) -> (10.685, 5.355, 1.57)
  line L552 (10.685, 9.885, 1.57) -> (10.685, 10.435, 1.57)
  line L553 (10.685, 3.535, 1.57) -> (10.685, 4.085, 1.57)
  line L554 (9.635, 10.435, 1.57) -> (9.635, 9.885, 1.57)
  line L555 (9.635, 5.355, 1.57) -> (9.635, 4.805, 1.57)
  line L556 (9.635, 5.355, 1.57) -> (10.685, 4.805, 1.57)
  line L557 (9.635, 10.435, 1.57) -> (10.685, 9.885, 1.57)
  line L558 (10.685, 3.535, 1.57) -> (9.635, 4.085, 1.57)
  line L559 (9.885, 5.355, 1.57) -> (9.885, 4.805, 1.57)
  line L560 (10.435, 3.535, 1.57) -> (10.435, 4.085, 1.57)
  line L561 (9.885, 10.435, 1.57) -> (9.885, 9.885, 1.57)
  line L562 (10.685, 4.085, 1.57) -> (9.635, 4.085, 1.57)
  line L563 (9.635, 4.805, 1.57) -> (10.685, 4.805, 1.57)
  line L564 (9.635, 9.885, 1.57) -> (10.685, 9.885, 1.57)
  line L565 (9.36, 11.78, 1.57) -> (9.36, 11.08, 1.57)
  line L566 (10.96, 7.27, 1.57) -> (10.96, 7.97, 1.57)
  line L567 (10.96, 6, 1.57) -> (10.96, 6.7, 1.57)
  line L568 (9.36, 13.05, 1.57) -> (9.36, 12.35, 1.57)
  line L569 (10.96, 8.54, 1.57) -> (10.96, 9.24, 1.57)
  line L570 (10.96, 16.16, 1.57) -> (10.96, 16.86, 1.57)
  line L571 (10.96, 13.62, 1.57) -> (10.96, 14.32, 1.57)
  line L572 (10.96, 14.89, 1.57) -> (10.96, 15.59, 1.57)
  line L573 (9.36, 15.59, 1.57) -> (9.36, 14.89, 1.57)
  line L574 (10.96, 12.35, 1.57) -> (10.96, 13.05, 1.57)
  line L575 (9.36, 9.24, 1.57) -> (9.36, 8.54, 1.57)
  line L576 (9.36, 7.97, 1.57) -> (9.36, 7.27, 1.57)
  line L577 (10.96, 11.08, 1.57) -> (10.96, 11.78, 1.57)
  line L578 (9.36, 6.7, 1.57) -> (9.36, 6, 1.57)
  line L579 (9.36, 16.86, 1.57) -> (9.36, 16.16, 1.57)
  line L580 (9.36, 14.32, 1.57) -> (9.36, 13.62, 1.57)
  line L581 (10.36, 6.7, 1.57) -> (10.36, 6, 1.57)
  line L582 (9.96, 11.08, 1.57) -> (9.96, 11.78, 1.57)
  line L583 (10.36, 14.32, 1.57) -> (10.36, 13.62, 1.57)
  line L584 (9.96, 12.35, 1.57) -> (9.96, 13.05, 1.57)
  line L585 (10.36, 9.24, 1.57) -> (10.36, 8.54, 1.57)
  line L586 (10.36, 7.97, 1.57) -> (10.36, 7.27, 1.57)
  line L587 (10.36, 16.86, 1.57) -> (10.36, 16.16, 1.57)
  line L588 (10.36, 15.59, 1.57) -> (10.36, 14.89, 1.57)
  line L589 (10.96, 11.78, 1.57) -> (10.36, 11.78, 1.57)
  line L590 (10.96, 13.05, 1.57) -> (10.36, 13.05, 1.57)
  line L591 (9.36, 8.54, 1.57) -> (9.96, 8.54, 1.57)
  line L592 (9.36, 7.27, 1.57) -> (9.96, 7.27, 1.57)
  line L593 (9.36, 6, 1.57) -> (9.96, 6, 1.57)
  line L594 (9.36, 13.62, 1.57) -> (9.96, 13.62, 1.57)
  line L595 (9.36, 16.16, 1.57) -> (9.96, 16.16, 1.57)
  line L596 (9.36, 14.89, 1.57) -> (9.96, 14.89, 1.57)
  line L597 (9.96, 11.78, 1.57) -> (9.36, 11.78, 1.57)
  line L598 (10.36, 8.54, 1.57) -> (10.96, 8.54, 1.57)
  line L599 (10.36, 6, 1.57) -> (10.96, 6, 1.57)
  line L600 (10.36, 7.27, 1.57) -> (10.96, 7.27, 1.57)
  line L601 (10.36, 13.62, 1.57) -> (10.96, 13.62, 1.57)
  line L602 (10.36, 16.16, 1.57) -> (10.96, 16.16, 1.57)
  line L603 (10.36, 14.89, 1.57) -> (10.96, 14.89, 1.57)
  line L604 (9.96, 13.05, 1.57) -> (9.36, 13.05, 1.57)
  line L605 (9.36, 12.35, 1.57) -> (9.96, 12.35, 1.57)
  line L606 (10.96, 14.32, 1.57) -> (10.36, 14.32, 1.57)
  line L607 (10.96, 9.24, 1.57) -> (10.36, 9.24, 1.57)
  line L608 (10.96, 15.59, 1.57) -> (10.36, 15.59, 1.57)
  line L609 (10.96, 7.97, 1.57) -> (10.36, 7.97, 1.57)
  line L610 (10.96, 6.7, 1.57) -> (10.36, 6.7, 1.57)
  line L611 (9.36, 11.08, 1.57) -> (9.96, 11.08, 1.57)
  line L612 (10.96, 16.86, 1.57) -> (10.36, 16.86, 1.57)
  line L613 (9.96, 9.24, 1.57) -> (9.36, 9.24, 1.57)
  line L614 (9.96, 6.7, 1.57) -> (9.36, 6.7, 1.57)
  line L615 (9.96, 16.86, 1.57) -> (9.36, 16.86, 1.57)
  line L616 (10.36, 11.08, 1.57) -> (10.96, 11.08, 1.57)
  line L617 (9.96, 7.97, 1.57) -> (9.36, 7.97, 1.57)
  line L618 (10.36, 12.35, 1.57) -> (10.96, 12.35, 1.57)
  line L619 (9.96, 14.32, 1.57) -> (9.36, 14.32, 1.57)
  line L620 (9.96, 15.59, 1.57) -> (9.36, 15.59, 1.57)
  line L621 (9.96, 7.27, 1.57) -> (9.96, 7.97, 1.57)
  line L622 (9.96, 8.54, 1.57) -> (9.96, 9.24, 1.57)
  line L623 (9.96, 13.62, 1.57) -> (9.96, 14.32, 1.57)
  line L624 (9.96, 16.16, 1.57) -> (9.96, 16.86, 1.57)
  line L625 (9.96, 14.89, 1.57) -> (9.96, 15.59, 1.57)
  line L626 (10.36, 11.78, 1.57) -> (10.36, 11.08, 1.57)
  line L627 (9.96, 6, 1.57) -> (9.96, 6.7, 1.57)
  line L628 (10.36, 13.05, 1.57) -> (10.36, 12.35, 1.57)
  line L629 (6.4362, 15.875, 1.57) -> (6.4362, 14.605, 1.57)
  line L630 (6.4362, 5.715, 1.57) -> (6.4362, 4.445, 1.57)
  line L631 (13.8838, 12.065, 1.57) -> (13.8838, 13.335, 1.57)
  line L632 (6.4362, 8.255, 1.57) -> (6.4362, 6.985, 1.57)
  line L633 (6.4362, 13.335, 1.57) -> (6.4362, 12.065, 1.57)
  line L634 (6.4362, 6.985, 1.57) -> (6.4362, 5.715, 1.57)
  line L635 (13.8838, 13.335, 1.57) -> (13.8838, 14.605, 1.57)
  line L636 (6.4362, 14.605, 1.57) -> (6.4362, 13.335, 1.57)
  line L637 (5.9655, 8.255, 1.57) -> (5.9655, 6.985, 1.57)
  line L638 (14.3545, 9.525, 1.57) -> (14.3545, 10.795, 1.57)
  line L639 (5.9655, 17.145, 1.57) -> (5.9655, 15.875, 1.57)
  line L640 (5.9655, 15.875, 1.57) -> (5.9655, 14.605, 1.57)
  line L641 (5.9655, 10.795, 1.57) -> (5.9655, 9.525, 1.57)
  line L642 (14.3545, 10.795, 1.57) -> (14.3545, 12.065, 1.57)
  line L643 (5.9655, 9.525, 1.57) -> (5.9655, 8.255, 1.57)
  line L644 (5.9655, 18.415, 1.57) -> (5.9655, 17.145, 1.57)
  line L645 (10.795, 5.715, 1.57) -> (6.4362, 5.715, 1.57)
  line L646 (9.525, 12.065, 1.57) -> (13.8838, 12.065, 1.57)
  line L647 (10.795, 15.875, 1.57) -> (6.4362, 15.875, 1.57)
  line L648 (10.795, 14.605, 1.57) -> (6.4362, 14.605, 1.57)
  line L649 (10.795, 13.335, 1.57) -> (6.4362, 13.335, 1.57)
  line L650 (9.525, 13.335, 1.57) -> (13.8838, 13.335, 1.57)
  line L651 (10.795, 6.985, 1.57) -> (6.4362, 6.985, 1.57)
  line L652 (10.795, 8.255, 1.57) -> (6.4362, 8.255, 1.57)
  line L653 (10.795, 6.985, 1.57) -> (10.795, 8.255, 1.57)
  line L654 (10.795, 9.525, 1.57) -> (10.795, 10.795, 1.57)
  line L655 (10.795, 15.875, 1.57) -> (10.795, 17.145, 1.57)
  line L656 (9.525, 10.795, 1.57) -> (9.525, 9.525, 1.57)
  line L657 (9.525, 12.065, 1.57) -> (9.525, 10.795, 1.57)
  line L658 (10.795, 8.255, 1.57) -> (10.795, 9.525, 1.57)
  line L659 (10.795, 14.605, 1.57) -> (10.795, 15.875, 1.57)
  line L660 (10.795, 17.145, 1.57) -> (10.795, 18.415, 1.57)
  line L661 (10.795, 4.445, 1.57) -> (10.795, 5.715, 1.57)
  line L662 (10.795, 14.605, 1.57) -> (10.795, 15.875, 1.57)
  line L663 (10.795, 5.715, 1.57) -> (10.795, 6.985, 1.57)
  line L664 (9.525, 13.335, 1.57) -> (9.525, 12.065, 1.57)
  line L665 (10.795, 12.065, 1.57) -> (10.795, 13.335, 1.57)
  line L666 (10.795, 6.985, 1.57) -> (10.795, 8.255, 1.57)
  line L667 (10.795, 13.335, 1.57) -> (10.795, 14.605, 1.57)
  line L668 (9.525, 14.605, 1.57) -> (9.525, 13.335, 1.57)
  line L669 (13.8838, 14.605, 1.57) -> (9.525, 14.605, 1.57)
  line L670 (6.4362, 12.065, 1.57) -> (10.795, 12.065, 1.57)
  line L671 (6.4362, 14.605, 1.57) -> (10.795, 14.605, 1.57)
  line L672 (6.4362, 4.445, 1.57) -> (10.795, 4.445, 1.57)
  line L673 (13.8838, 13.335, 1.57) -> (9.525, 13.335, 1.57)
  line L674 (6.4362, 6.985, 1.57) -> (10.795, 6.985, 1.57)
  line L675 (6.4362, 5.715, 1.57) -> (10.795, 5.715, 1.57)
  line L676 (6.4362, 13.335, 1.57) -> (10.795, 13.335, 1.57)
  line L677 (10.795, 10.795, 1.57) -> (5.9655, 10.795, 1.57)
  line L678 (10.795, 17.145, 1.57) -> (5.9655, 17.145, 1.57)
  line L679 (9.525, 10.795, 1.57) -> (14.3545, 10.795, 1.57)
  line L680 (10.795, 9.525, 1.57) -> (5.9655, 9.525, 1.57)
  line L681 (10.795, 15.875, 1.57) -> (5.9655, 15.875, 1.57)
  line L682 (10.795, 18.415, 1.57) -> (5.9655, 18.415, 1.57)
  line L683 (9.525, 9.525, 1.57) -> (14.3545, 9.525, 1.57)
  line L684 (10.795, 8.255, 1.57) -> (5.9655, 8.255, 1.57)
  line L685 (14.3545, 12.065, 1.57) -> (9.525, 12.065, 1.57)
  line L686 (5.9655, 6.985, 1.57) -> (10.795, 6.985, 1.57)
  line L687 (14.3545, 10.795, 1.57) -> (9.525, 10.795, 1.57)
  line L688 (5.9655, 15.875, 1.57) -> (10.795, 15.875, 1.57)
  line L689 (5.9655, 9.525, 1.57) -> (10.795, 9.525, 1.57)
  line L690 (5.9655, 17.145, 1.57) -> (10.795, 17.145, 1.57)
  line L691 (5.9655, 14.605, 1.57) -> (10.795, 14.605, 1.57)
  line L692 (5.9655, 8.255, 1.57) -> (10.795, 8.255, 1.57)
  line L693 (3.8971, 4.5799, 1.57) -> (6.007, 4.5799, 1.57)
  line L694 (3.8971, 17.2799, 1.57) -> (6.007, 17.2799, 1.57)
  line L695 (3.8971, 4.5799, 1.57) -> (3.8971, 3.0401, 1.57)
  line L696 (3.8971, 17.2799, 1.57) -> (3.8971, 15.7401, 1.57)
  line L697 (3.8971, 3.0401, 1.57) -> (6.007, 3.0401, 1.57)
  line L698 (3.8971, 15.7401, 1.57) -> (6.007, 15.7401, 1.57)
  line L699 (6.2629, 3.3541, 1.57) -> (6.2629, 4.2659, 1.57)
  line L700 (6.2629, 16.0541, 1.57) -> (6.2629, 16.9659, 1.57)
  line L701 (4.7629, 3.3541, 1.57) -> (4.7629, 4.2659, 1.57)
  line L702 (4.7629, 16.0541, 1.57) -> (4.7629, 16.9659, 1.57)
  line L703 (5.6511, 16.0541, 1.57) -> (6.2629, 16.0541, 1.57)
  line L704 (5.6511, 3.3541, 1.57) -> (6.2629, 3.3541, 1.57)
  line L705 (4.1511, 3.3541, 1.57) -> (4.7629, 3.3541, 1.57)
  line L706 (4.1511, 16.0541, 1.57) -> (4.7629, 16.0541, 1.57)
  line L707 (6.2629, 16.9659, 1.57) -> (5.6511, 16.9659, 1.57)
  line L708 (6.2629, 4.2659, 1.57) -> (5.6511, 4.2659, 1.57)
  line L709 (4.1511, 4.2659, 1.57) -> (4.1511, 3.3541, 1.57)
  line L710 (4.1511, 16.9659, 1.57) -> (4.1511, 16.0541, 1.57)
  line L711 (4.7629, 4.2659, 1.57) -> (4.1511, 4.2659, 1.57)
  line L712 (4.7629, 16.9659, 1.57) -> (4.1511, 16.9659, 1.57)
  line L713 (5.6511, 4.2659, 1.57) -> (5.6511, 3.3541, 1.57)
  line L714 (5.6511, 16.9659, 1.57) -> (5.6511, 16.0541, 1.57)
  line L715 (7.4644, 2.4051, 1.57) -> (2.6956, 2.4051, 1.57)
  line L716 (7.4644, 15.1051, 1.57) -> (2.6956, 15.1051, 1.57)